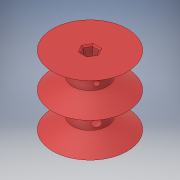
# Autodesk Inventor part: spoolV06
Saved by Autodesk Inventor 2019.4 (Build 234330000, 330)
## iProperties
Created: 2019-02-25
Part Number: spoolV06
Material: PC/ABS Plastic
Document SubType Name: Modeling
Designer: steele
Density: 0.357273 g/cm^3
Appearance: Smooth - Red
holeForString: 0.200 in
stringDiameter: 0.120 in
clearanceForString: 0.080 in
clearanceForHexShaft: 0.023 in
hexDiameter: 0.523 in
supportChannels: 0.150 in
spoolInteriorDiameter: 1.500 in
spoolInteriroRadius: 0.750 in
spoolExteriorDiameter: 3.250 in
spoolExteriorRadius: 1.625 in
spoolFiletRadius: 0.075 in
holeCenter: 0.575 in
hexHoleChamfer: 0.063 in
stringHoleCenterFromHexShaft: 0.361 in
textCircleDiameter: 2.438 in
textHeight: 0.240 in
textDepth: 0.050 in
stringHoleChamfer: 0.188 in
spoolTotalHeight: 3.000 in
spaceHeight: 0.250 in
spacerDiameter: 0.950 in
spoolHeightWithoutSpacer: 2.750 in
d100: 0.063 in
Author: steele
Autodesk Inventor part; units mm, degrees
ref_plane "XZ Plane" through (0, 0, 0) normal (0, 1, 0) x (-1, 0, 0)
ref_plane "XY Plane" through (0, 0, 0) normal (0, 0, 1) x (1, 0, 0)
sketch "Sketch15" plane through (0, 0, 0) normal (0, 0, 1) x (1, 0, 0)
  line L0 (41.275, 0) -> (41.275, 76.2) construction
  line L1 (0, 0) -> (41.275, 0)
  line L2 (0, 76.2) -> (41.275, 76.2)
  line L3 (19.05, 0) -> (19.05, 76.2) construction
  line L4 (0, 76.2) -> (0, 0)
  line L5 (19.05, 19.05) -> (41.275, 19.05) construction
  line L6 (41.275, 0) -> (19.05, 12.8316)
  line L7 (41.275, 38.1) -> (19.05, 25.2684)
  line L8 (19.05, 25.2684) -> (41.275, 25.2684) construction
  line L9 (19.05, 25.2684) -> (19.05, 12.8316)
  line L10 (41.275, 38.1) -> (19.05, 50.9316)
  line L11 (19.05, 50.9316) -> (19.05, 63.3684)
  line L12 (19.05, 63.3684) -> (41.275, 76.2)
  line L13 (41.275, 38.1) -> (19.05, 38.1) construction
  line L14 (19.05, 63.3684) -> (41.275, 63.3684) construction
  dimension "d85" = 41.275
  dimension "d86" = 76.2
  dimension "d87" = 19.05
  dimension "d88" = 41.275
  dimension "d89" = 38.1
  dimension "centerLineForSpool" = 19.05
  dimension "d93" = 30
  dimension "d94" = 30
  dimension "d95" = 30
  dimension "d96" = 30
  constraints: 30 end point, 10 point on line, 3 horizontal, 2 midpoint, 2 perpendicular, 1 collinear, 1 parallel, 1 vertical
  measures "d85" distance from line of L1.start L0
  measures "d86" distance of L0.start L0.end
  measures "d87" distance from line of L3 L1.start
  measures "d88" distance of L2.start L0.end
  measures "d89" distance from line of L7.start L1
  measures "centerLineForSpool" distance from line of L5.start L1
  measures "d93" angle of L6 L1
  measures "d94" angle of L7 L8
  measures "d95" angle of L10 L13
  measures "d96" angle of L12 L14
revolve "Revolution2" add sketch "Sketch15" angle 360 about axis through (0, 76.2, 0) along (0, -1, 0)
sketch "Sketch16" plane through (0, 0, 0) normal (0, -1, 0) x (1, 0, 0)
  line L0 (-7.6623, 0) -> (-3.8312, 6.6357)
  line L1 (-3.8312, 6.6357) -> (3.8312, 6.6357)
  line L2 (3.8312, 6.6357) -> (7.6623, 0)
  line L3 (7.6623, 0) -> (3.8312, -6.6358)
  line L4 (3.8312, -6.6358) -> (-3.8312, -6.6358)
  line L5 (-3.8312, -6.6358) -> (-7.6623, 0)
  point P0 (0, 0)
  point P1 (0, 0)
  dimension "d103" = 13.2715
  constraints: 12 end point, 1 coincident, 1 horizontal, 13 other
  measures "d103" distance between parallel lines of L1 L4
extrude "Extrusion11" cut sketch "Sketch16" against normal through all
sketch "Sketch17" plane through (0, 0, 0) normal (1, 0, 0) x (0, 1, 0)
  circle A0 centre (57.15, 9.1757) radius 2.54
  circle A1 centre (19.05, 9.1757) radius 2.54
  line L0 (0, 41.275) -> (0, -41.275) projected
  line L1 (76.2, 41.275) -> (76.2, -41.275) projected
  line L2 (0, 6.6357) -> (76.2, 6.6357) projected
  point P0 (0, 0)
  dimension "d110" = 19.05
  dimension "d111" = 19.05
  dimension "d112" = 5.08
  constraints: 2 centre point, 2 tangent, 1 equal radius
  measures "d110" distance from line of A1.centre L0
  measures "d111" distance from line of A0.centre L1
  measures "d112" diameter of A0
extrude "Extrusion13" cut sketch "Sketch17" along normal through all both and the other way through all
ref_plane "Work Plane4" through (-19.05, 0, 0) normal (1, 0, 0) x (0, 1, 0)
sketch "Sketch22" plane through (-19.05, 0, 0) normal (1, 0, 0) x (0, 1, 0)
  spline S0 degree 8 poles (59.69, 9.1757) (59.69, 9.4517) (59.6557, 9.7212) (59.59, 9.9804) (59.4956, 10.2261) (59.3755, 10.4557) (59.2323, 10.6669) (59.0691, 10.858) (58.7144, 11.191) (58.5225, 11.336) (58.3154, 11.4599) (58.0958, 11.5609) (57.8667, 11.6378) (57.6308, 11.6896) (57.3909, 11.7157) (56.8686, 11.7157) (56.5893, 11.6801) (56.3163, 11.6098) (56.0539, 11.5059) (55.8062, 11.37) (55.5775, 11.2041) (55.3719, 11.0111) (55.0147, 10.5794) (54.8595, 10.3366) (54.7333, 10.0693) (54.6415, 9.7817) (54.5882, 9.479) (54.5771, 9.1672) (54.6105, 8.8531) (54.8032, 8.1024) (55.0034, 7.6991) (55.2751, 7.3483) (55.6037, 7.0608) (55.9729, 6.8444) (56.3656, 6.703) (56.7635, 6.6357) (57.4276, 6.6357) (57.7065, 6.6704) (57.9827, 6.7403) (58.2517, 6.8459) (58.509, 6.9871) (58.7494, 7.1637) (58.9676, 7.3748) (59.2832, 7.7816) (59.3962, 7.9584) (59.4932, 8.1474) (59.5721, 8.3459) (59.6315, 8.5511) (59.6708, 8.76) (59.69, 8.9692) (59.69, 9.1757) knots 0 0 0 0 0 0 0 0 0 0.129052 0.129052 0.129052 0.129052 0.129052 0.129052 0.129052 0.253777 0.253777 0.253777 0.253777 0.253777 0.253777 0.253777 0.399469 0.399469 0.399469 0.399469 0.399469 0.399469 0.399469 0.544533 0.544533 0.544533 0.544533 0.544533 0.544533 0.544533 0.751894 0.751894 0.751894 0.751894 0.751894 0.751894 0.751894 0.900801 0.900801 0.900801 0.900801 0.900801 0.900801 0.900801 1 1 1 1 1 1 1 1 1 projected
  circle A0 centre (57.15, 9.1757) radius 3.9688
  circle A1 centre (57.15, 9.1757) radius 2.54 construction
  line L0 (57.15, 6.6357) -> (76.2, 6.6357) construction
  line L1 (76.2, 41.275) -> (76.2, -41.275) construction
  point P0 (0, 0)
  dimension "d121" = 19.05
  dimension "d122" = 5.08
  dimension "d125" = 7.9375
  constraints: 2 centre point, 1 concentric, 1 tangent, 1 vertical alignment
  measures "d121" distance from line of A1.centre L1
  measures "d122" diameter of A1
  measures "d125" diameter of A0
extrude "Extrusion16" cut sketch "Sketch22" along normal blind 11.1125
ref_plane "Work Plane5" through (19.05, 0, 0) normal (1, 0, 0) x (0, 1, 0)
sketch "Sketch23" plane through (19.05, 0, 0) normal (1, 0, 0) x (0, 1, 0)
  line L0 (19.05, 6.6357) -> (57.15, 6.6357) projected
  circle A0 centre (19.05, 9.1757) radius 2.54 construction
  line L1 (0, 41.275) -> (0, -41.275) projected
  circle A1 centre (19.05, 9.1757) radius 3.9688
  point P0 (0, 0)
  dimension "d127" = 5.08
  dimension "d128" = 19.05
  dimension "d129" = 7.9375
  constraints: 2 centre point, 1 coincident, 1 tangent
  measures "d127" diameter of A0
  measures "d128" distance from line of A0.centre L1
  measures "d129" diameter of A1
extrude "Extrusion17" cut sketch "Sketch23" against normal blind 11.1125
chamfer "Chamfer10" distance 1.5875 angle 45 12 edges at (0, 76.2, -6.6358) (5.7467, 76.2, -3.3179) (5.7467, 76.2, 3.3179) (0, 76.2, 6.6357) (-5.7467, 76.2, 3.3179) (-5.7467, 76.2, -3.3179) (-5.7467, 0, -3.3179) (-5.7467, 0, 3.3179) (0, 0, 6.6357) (5.7467, 0, 3.3179) (5.7467, 0, -3.3179) (0, 0, -6.6358)
equation "\"d85\" = spoolExteriorRadius"
equation "\"d86\" = spoolOverallHeight"
equation "\"d88\" = d85"
equation "\"d89\" = 0.5 * spoolOverallHeight"
equation "\"centerLineForSpool\" = 0.25 * spoolOverallHeight"
equation "\"d103\" = hexDiameter"
equation "\"d110\" = centerLineForSpool"
equation "\"d111\" = centerLineForSpool"
equation "\"d112\" = holeForString"
equation "\"d121\" = centerLineForSpool"
equation "\"d122\" = holeForString"
equation "\"d125\" = knotHoleDiameter"
equation "\"d127\" = holeForString"
equation "\"d128\" = centerLineForSpool"
equation "\"d129\" = knotHoleDiameter"
equation "\"d130\" = knotHoleDepth"
equation "\"d132\" = hexHoleChamfer"
equation "\"holeForString\" = stringDiameter + clearanceForString"
equation "\"stringDiameter\" = 3.048"
equation "\"clearanceForString\" = 2.032"
equation "\"spoolHeightWithoutSpacer\" = 69.85"
equation "\"hexShaftDiameter\" = 12.7"
equation "\"clearanceForHexShaft\" = 0.5715"
equation "\"hexDiameter\" = hexShaftDiameter + clearanceForHexShaft"
equation "\"supportChannels\" = 3.81"
equation "\"spoolInteriorDiameter\" = 38.1"
equation "\"spoolInteriroRadius\" = 0.5 * spoolInteriorDiameter"
equation "\"spoolExteriorDiameter\" = 82.55"
equation "\"spoolExteriorRadius\" = 0.5 * spoolExteriorDiameter"
equation "\"spoolFiletRadius\" = 0.5 * supportChannels"
equation "\"holeCenter\" = 0.25 * spoolHeightWithoutSpacer - 0.75 * supportChannels"
equation "\"hexHoleChamfer\" = 1.5875"
equation "\"stringHoleCenterFromHexShaft\" = 0.5 * hexDiameter + 0.5 * holeForString"
equation "\"textCircleDiameter\" = 0.75 * spoolExteriorDiameter"
equation "\"textHeight\" = 6.096"
equation "\"textDepth\" = 1.27"
equation "\"stringHoleChamfer\" = 4.7625"
equation "\"spoolTotalHeight\" = 76.2"
equation "\"spaceHeight\" = spoolTotalHeight - spoolHeightWithoutSpacer"
equation "\"spacerDiameter\" = 24.13"
equation "\"spoolOverallHeight\" = 76.2"
equation "\"d114\" = -spoolInteriroRadius"
equation "\"knotHoleDiameter\" = 7.9375"
equation "\"d126\" = spoolInteriroRadius"
equation "\"knotHoleDepth\" = 11.1125"
body "Solid3"
